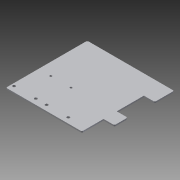
# Autodesk Inventor part: Mounting Board 3
Saved by Autodesk Inventor 2013 (Build 170138000, 138)
## iProperties
Created: 2013-01-26
Part Number: Mounting Board 3
Material: Aluminum 6061
Document SubType Name: Modeling
Designer: Moses
Mass: 278.804 g
Surface Area: 677.515 cm^2
Volume: 102.88 cm^3
Density: 2.71 g/cm^3
Author: Moses
Autodesk Inventor part; units mm, degrees
ref_plane "YZ Plane" through (0, 0, 0) normal (1, 0, 0) x (0, 1, 0)
ref_plane "XZ Plane" through (0, 0, 0) normal (0, 1, 0) x (-1, 0, 0)
ref_plane "XY Plane" through (0, 0, 0) normal (0, 0, 1) x (1, 0, 0)
sketch "Sketch1" plane through (0, 0, 0) normal (0, 1, 0) x (-1, 0, 0)
  line L0 (0, 0) -> (203.2, 0)
  line L1 (203.2, 0) -> (203.2, 152.4)
  line L2 (203.2, 152.4) -> (0, 152.4)
  line L3 (0, 152.4) -> (0, 0)
  line L4 (127, 101.6) -> (174.244, 101.6) construction
  circle A0 centre (127, 101.6) radius 2.54
  circle A1 centre (174.244, 101.6) radius 2.54
  circle A2 centre (12.7, 139.7) radius 3.302 construction
  circle A3 centre (12.7, 165.1) radius 3.302 construction
  arc A4 (0, 128.5875) -> (1.5875, 127) centre (1.5875, 128.5875) ccw construction
  line L5 (1.5875, 127) -> (23.8125, 127) construction
  arc A5 (23.8125, 127) -> (25.4, 128.5875) centre (23.8125, 128.5875) ccw construction
  line L6 (25.4, 128.5875) -> (25.4, 176.2125) construction
  arc A6 (25.4, 176.2125) -> (23.8125, 177.8) centre (23.8125, 176.2125) ccw construction
  line L7 (23.8125, 177.8) -> (1.5875, 177.8) construction
  arc A7 (1.5875, 177.8) -> (0, 176.2125) centre (1.5875, 176.2125) ccw construction
  line L8 (0, 176.2125) -> (0, 128.5875) construction
  circle A8 centre (12.7, 86.5011) radius 3.302 construction
  circle A9 centre (12.7, 42.0511) radius 3.302 construction
  line L9 (25.4, 96.0261) -> (25.4, 32.5261) construction
  line L10 (25.4, 32.5261) -> (0, 32.5261) construction
  line L11 (0, 96.0261) -> (0, 32.5261) construction
  line L12 (25.4, 96.0261) -> (0, 96.0261) construction
  line L13 (0, 96.0261) -> (25.4, 96.0261)
  line L14 (25.4, 96.0261) -> (25.4, 32.5261)
  line L15 (0, 32.5261) -> (25.4, 32.5261)
  line L16 (0, 127) -> (25.4, 127)
  line L17 (25.4, 152.4) -> (25.4, 127)
  line L18 (0, 96.0261) -> (0, 32.5261)
  line L19 (0, 127) -> (0, 152.4)
  line L20 (0, 152.4) -> (25.4, 152.4)
  line L21 (203.2, 152.4) -> (203.2, 177.8)
  line L22 (25.4, 152.4) -> (25.4, 177.8)
  line L23 (25.4, 177.8) -> (203.2, 177.8)
  circle A10 centre (69.85, 165.1) radius 3.302 projected
  circle A11 centre (196.85, 165.1) radius 3.302 projected
  circle A12 centre (146.05, 165.1) radius 3.302 projected
  circle A13 centre (120.65, 165.1) radius 3.302 projected
  line L24 (0, 0) -> (0, -12.7)
  line L25 (0, -12.7) -> (203.2, -12.7)
  line L26 (203.2, -12.7) -> (203.2, 0)
  dimension "d0" = 203.2
  dimension "d2" = 152.4
  dimension "d8" = 47.244
  dimension "d9" = 5.08
  dimension "d10" = 101.6
  dimension "d11" = 127
  dimension "d17" = 25.4
  dimension "d19" = 12.7
  constraints: 38 end point, 6 perpendicular, 5 parallel, 5 point on line, 4 collinear, 2 centre point, 2 coincident, 1 equal radius, 1 horizontal, 1 midpoint
  measures "d0" distance of L1.end L2.end
  measures "d2" distance of L0.end L1.end
  measures "d8" distance of L4.start L4.end
  measures "d9" diameter of A0
  measures "d10" distance between parallel lines of L0 L4
  measures "d11" distance from line of L4.start L3
  measures "d17" distance of L1.end L21.end
  measures "d19" distance of L0.start L24.end
extrude "Extrusion1" add sketch "Sketch1" along normal blind 3.175 contours L3 L15 L14 L13 L16 L17 L2 L1 L0 | L0 L26 L25 L24 | L2 L22 L23 L21
fillet "Fillet1" radius 3.175 7 edges at (-203.2, 1.5875, -12.7) (0, 1.5875, -12.7) (0, 1.5875, 32.5261) (0, 1.5875, 96.0261) (0, 1.5875, 127) (-25.4, 1.5875, 177.8) (-203.2, 1.5875, 177.8)
body "Solid1"
